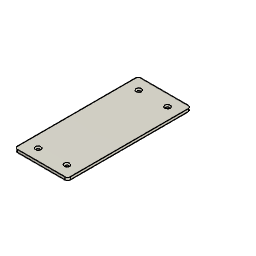
Dual 4020 Fan Hat - BLANK Platform (Autodesk Fusion 360 design; units mm, degrees)
Autodesk Fusion 360 part; units mm, degrees
sketch "Sketch1" plane through (0, 0, 66) normal (0, 0, 1) x (-1, 0, 0)
  circle A0 centre (16.3, -57) radius 1.425
  circle A1 centre (16.3, 57) radius 1.425
  circle A2 centre (-16.3, -57) radius 1.425
  circle A3 centre (-16.3, 57) radius 1.425
  arc A4 (-19.3, -50.4) -> (-22.3, -53.4) centre (-19.3, -53.4) ccw
  line L0 (-22.3, -53.4) -> (-22.3, -60.6)
  arc A5 (-22.3, -60.6) -> (-19.3, -63.6) centre (-19.3, -60.6) ccw
  line L1 (-19.3, -63.6) -> (19.3, -63.6)
  arc A6 (19.3, -63.6) -> (22.3, -60.6) centre (19.3, -60.6) ccw
  line L2 (22.3, -60.6) -> (22.3, -53.4)
  arc A7 (22.3, -53.4) -> (19.3, -50.4) centre (19.3, -53.4) ccw
  line L3 (19.3, -50.4) -> (16.3, -50.4)
  line L4 (16.3, -50.4) -> (16.3, 50.4)
  line L5 (16.3, 50.4) -> (19.3, 50.4)
  arc A8 (19.3, 50.4) -> (22.3, 53.4) centre (19.3, 53.4) ccw
  line L6 (22.3, 53.4) -> (22.3, 60.6)
  arc A9 (22.3, 60.6) -> (19.3, 63.6) centre (19.3, 60.6) ccw
  line L7 (19.3, 63.6) -> (-19.3, 63.6)
  arc A10 (-19.3, 63.6) -> (-22.3, 60.6) centre (-19.3, 60.6) ccw
  line L8 (-22.3, 60.6) -> (-22.3, 53.4)
  arc A11 (-22.3, 53.4) -> (-19.3, 50.4) centre (-19.3, 53.4) ccw
  line L9 (-19.3, 50.4) -> (-16.3, 50.4)
  line L10 (-16.3, 50.4) -> (-16.3, -50.4)
  line L11 (-16.3, -50.4) -> (-19.3, -50.4)
  line L12 (-13.3, -50.4) -> (-13.3, 50.4)
  arc A12 (-7.1, 56.6) -> (-13.3, 50.4) centre (-7.1, 50.4) ccw
  line L13 (-7.1, 56.6) -> (7.1, 56.6)
  arc A13 (13.3, 50.4) -> (7.1, 56.6) centre (7.1, 50.4) ccw
  line L14 (13.3, 50.4) -> (13.3, -50.4)
  arc A14 (7.1, -56.6) -> (13.3, -50.4) centre (7.1, -50.4) ccw
  line L15 (7.1, -56.6) -> (-7.1, -56.6)
  arc A15 (-13.3, -50.4) -> (-7.1, -56.6) centre (-7.1, -50.4) ccw
  line L16 (-30, -70) -> (30, -70)
  line L17 (30, -70) -> (30, 70)
  line L18 (30, 70) -> (-30, 70)
  line L19 (-30, 70) -> (-30, -70)
  line L20 (0, -119.4716) -> (0, -115.6118)
  line L21 (0, -115.6118) -> (0, 115.6118) construction
  line L22 (-65.0661, 0) -> (-62.8605, 0)
  line L23 (-62.8605, 0) -> (62.8605, 0) construction
  point P0 (0, -70)
  point P1 (-30, 0)
  dimension "d139" = 60
  dimension "d140" = 140
  constraint horizontal L16
  constraint vertical L17
  constraint horizontal L18
  constraint vertical L19
  constraint parallel L0 L20
  constraint parallel L0 L21
  constraint midpoint origin L21
  constraint horizontal L22
  constraint parallel L22 L23
  constraint midpoint origin L23
  constraint midpoint L16 P0
  constraint midpoint L19 P1
  constraint horizontal origin P1
  constraint vertical origin P0
  measures "d139" distance of L16.start L16.end
  measures "d140" distance of L16.start L18.end
extrude "Extrude1" add sketch "Sketch1" along normal blind 3 contours A4 L0 A5 L1 A6 L2 A7 L3 L4 L5 A8 L6 A9 L7 A10 L8 A11 L9 L10 L11 | L12 A12 L13 A13 L14 A14 L15 A15 | L16 L17 L18 L19
sketch "Sketch2" plane through (0, 0, 69) normal (0, 0, 1) x (-1, 0, 0)
  circle A0 centre (-16.3, 57) radius 1.425
  circle A1 centre (16.3, 57) radius 1.425
  circle A2 centre (16.3, -57) radius 1.425
  circle A3 centre (-16.3, -57) radius 1.425
  line L0 (-30, 70) -> (-30, -70)
  line L1 (-30, -70) -> (30, -70)
  line L2 (30, -70) -> (30, 70)
  line L3 (30, 70) -> (-30, 70)
  circle A4 centre (-16.3, -57) radius 1.6
  circle A5 centre (16.3, -57) radius 1.6
  circle A6 centre (16.3, 57) radius 1.6
  circle A7 centre (-16.3, 57) radius 1.6
  dimension "d143" = 3.2
  dimension "d144" = 3.2
  dimension "d145" = 3.2
  dimension "d146" = 3.2
  constraint concentric A3 A4
  constraint concentric A2 A5
  constraint concentric A1 A6
  constraint concentric A0 A7
  measures "d143" diameter of A4
  measures "d144" diameter of A5
  measures "d145" diameter of A6
  measures "d146" diameter of A7
extrude "Extrude3" cut sketch "Sketch2" against normal blind 3 contours A4 | A5 | A6 | A7
chamfer "Chamfer1" distance 1.4 angle 45 4 edges at (-14.8083, 56.4214, 69) (17.7917, 56.4214, 69) (17.7917, -57.5786, 69) (-14.8083, -57.5786, 69)
fillet "Fillet1" radius 3 4 edges at (-30, -70, 67.5) (30, -70, 67.5) (-30, 70, 67.5) (30, 70, 67.5)
